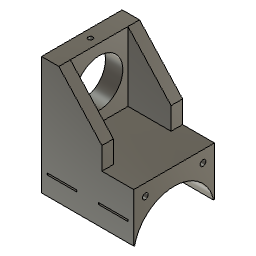
clutch holder v8 (Autodesk Fusion 360 design; units mm, degrees)
Autodesk Fusion 360 part; units mm, degrees
sketch "Sketch1" plane through (0, 0, 0) normal (0, 0, 1) x (1, 0, 0)
  line L0 (0, 0) -> (140, 0)
  line L1 (140, 0) -> (140, 140)
  line L2 (140, 140) -> (0, 140)
  line L3 (0, 140) -> (0, 0)
  line L4 (0, 140) -> (50, 140)
  line L5 (50, 140) -> (50, 0)
  line L6 (50, 0) -> (0, 0)
  line L7 (0, 0) -> (0, 140)
  dimension "d1" = 140
  dimension "d2" = 140
  constraint horizontal L0
  constraint vertical L1
  constraint horizontal L2
  constraint vertical L3
  constraint coincident L0.start L3.end
  constraint horizontal L4
  constraint vertical L5
  constraint horizontal L6
  constraint vertical L7
  constraint coincident L0 L5.end
  measures "d1" distance of L0.start L2.end
  measures "d2" distance of L0.start L0.end
extrude "Extrude1" add sketch "Sketch1" along normal blind 20 contours L0 L1 L2 L5 makes body 1
extrude "Extrude2" add sketch "Sketch1" along normal blind 140 contours L0 L2 L3 L4 L5 L6 L7 bodies 1
sketch "Sketch2" plane through (0, 0, 0) normal (-1, 0, 0) x (0, -1, 0)
  line L0 (-140, 0) -> (0, 0)
  line L1 (0, 0) -> (0, 140)
  line L2 (0, 140) -> (-140, 140)
  line L3 (-140, 140) -> (-140, 0)
  circle A0 centre (-70, 80) radius 41
  circle A1 centre (-70, 80) radius 51
  dimension "d7" = 82
  dimension "d8" = 102
  constraint concentric A0 A1
  measures "d7" diameter of A0
  measures "d8" diameter of A1
extrude "Extrude3" cut sketch "Sketch2" against normal blind 100 contours A0 bodies 1
sketch "Sketch3" plane through (0, 0, 20) normal (0, 0, 1) x (-1, 0, 0)
  line L0 (-50, -140) -> (-50, 0)
  line L1 (-50, 0) -> (-140, 0)
  line L2 (-140, 0) -> (-140, -140)
  line L3 (-140, -140) -> (-50, -140)
sketch "Sketch4" plane through (50, 0, 0) normal (1, 0, 0) x (0, 1, 0)
  circle A0 centre (70, 80) radius 41
  line L0 (0, 20) -> (140, 20)
  line L1 (140, 20) -> (140, 140)
  line L2 (140, 140) -> (0, 140)
  line L3 (0, 140) -> (0, 20)
extrude "Extrude4" cut sketch "Sketch4" against normal blind 20 bodies 1
sketch "Sketch5" plane through (0, 0, 0) normal (0, -1, 0) x (1, 0, 0)
  line L0 (30, 20) -> (30, 140)
  line L1 (30, 140) -> (0, 140)
  line L2 (0, 140) -> (0, 0)
  line L3 (0, 0) -> (140, 0)
  line L4 (140, 0) -> (140, 20)
  line L5 (140, 20) -> (30, 20)
  line L6 (30, 20) -> (30, 140)
  line L7 (140, 20) -> (30, 20)
  line L8 (30, 140) -> (140, 20)
  constraint coincident L0.end L1.start
  constraint coincident L4.end L5.start
extrude "Extrude5" add sketch "Sketch5" against normal blind 20 contours L0 L5 L6 L7 L8 bodies 1
sketch "Sketch6" plane through (0, 140, 0) normal (0, 1, 0) x (-1, 0, 0)
  line L0 (-30, 140) -> (-30, 20)
  line L1 (-30, 20) -> (-140, 20)
  line L2 (-140, 20) -> (-140, 0)
  line L3 (-140, 0) -> (0, 0)
  line L4 (0, 0) -> (0, 140)
  line L5 (0, 140) -> (-30, 140)
  line L6 (-30, 140) -> (-30, 20)
  line L7 (-140, 20) -> (-50, 20)
  line L8 (-30, 140) -> (-140, 20)
  constraint coincident L0.start L5.end
  constraint coincident L1.end L2.start
extrude "Extrude6" add sketch "Sketch6" against normal blind 20 contours L0 L1 L6 L7 L8 bodies 1
sketch "Sketch7" plane through (0, 0, 0) normal (-1, 0, 0) x (0, -1, 0)
  line L0 (-70, 80) -> (-70, 58.5)
  dimension "d17" = 21.5
  constraint vertical L0
  measures "d17" distance of L0.start L0.end
sketch "Sketch8" plane through (0, 120, 0) normal (0, -1, 0) x (1, 0, 0)
  line L0 (30, 140) -> (30, 20)
  line L1 (30, 20) -> (140, 20)
  line L2 (140, 20) -> (30, 140)
sketch "Sketch9" plane through (0, 0, 20) normal (0, 0, 1) x (-1, 0, 0)
sketch "Sketch10" plane through (0, 120, 0) normal (0, -1, 0) x (1, 0, 0)
  line L0 (104.5688, 58.4811) -> (30, 58.4811)
  line L1 (30, 58.4811) -> (30, 48.4811)
  line L2 (30, 48.4811) -> (104.5688, 48.4811)
  line L3 (104.5688, 48.4811) -> (104.5688, 58.4811)
  dimension "d18" = 10
  constraint horizontal L0
  constraint vertical L1
  constraint horizontal L2
  constraint vertical L3
  measures "d18" distance of L0.start L2.end
extrude "Extrude7" add sketch "Sketch10" along normal blind 100 bodies 1
sketch "Sketch11" plane through (104.5688, 0, 0) normal (1, 0, 0) x (0, 1, 0)
  line L0 (120, 48.4811) -> (120, 58.4811)
  line L1 (120, 58.4811) -> (20, 58.4811)
  line L2 (20, 58.4811) -> (20, 48.4811)
  line L3 (20, 48.4811) -> (120, 48.4811)
  line L4 (20, 58.4811) -> (120, 58.4811)
  line L5 (120, 58.4811) -> (120, 48.4811)
  line L6 (120, 48.4811) -> (20, 48.4811)
  line L7 (20, 48.4811) -> (20, 58.4811)
  constraint horizontal L4
  constraint vertical L5
  constraint horizontal L6
  constraint vertical L7
  constraint coincident L0.start L3.end
  constraint coincident L1.end L2.start
extrude "Extrude8" add sketch "Sketch11" along normal blind 100 bodies 1
move_face "MoveFace1" by (30, 0, 0) 1 faces at (138.0067, 86.6667, 58.4811) on bodies 1
move_face "MoveFace2" by (10, 0, 0) 1 faces at (138.0067, 86.6667, 58.4811) on bodies 1
sketch "Sketch12" plane through (0, 0, 58.4811) normal (0, 0, 1) x (-1, 0, 0)
  line L0 (-104.7257, -120) -> (-30, -120)
  line L1 (-30, -120) -> (-30, -104.8989)
  line L2 (-30, -104.8989) -> (-30, -35.1011)
  line L3 (-30, -35.1011) -> (-30, -20)
  line L4 (-30, -20) -> (-104.7257, -20)
  line L5 (-104.7257, -20) -> (-204.5688, -20)
  line L6 (-204.5688, -20) -> (-204.5688, -120)
  line L7 (-204.5688, -120) -> (-104.7257, -120)
  line L8 (-140, -20) -> (-30, -20)
  line L9 (-30, -20) -> (-30, -120)
  line L10 (-30, -120) -> (-140, -120)
  line L11 (-140, -120) -> (-140, -20)
  constraint horizontal L8
  constraint vertical L9
  constraint horizontal L10
  constraint vertical L11
  constraint coincident L0.end L1.start
  constraint coincident L5 L8.start
extrude "Extrude9" cut sketch "Sketch12" against normal blind 20 contours L0 L1 L2 L3 L4 L5 L7 L8 L9 L10 L11 bodies 1 makes body 2 at (161.5229, 86.6667, 48.4811)
sketch "Sketch13" plane through (0, 0, 20) normal (0, 0, 1) x (-1, 0, 0)
  line L0 (-140, 0) -> (-240, 0)
  line L1 (-240, 0) -> (-240, -140)
  line L2 (-240, -140) -> (-140, -140)
  line L3 (-140, -140) -> (-140, 0)
  constraint horizontal L0
  constraint vertical L1
  constraint horizontal L2
  constraint vertical L3
extrude "Extrude10" add sketch "Sketch13" along normal blind 38.5 bodies 1 2
extrude "Extrude11" add 1 faces at (206.6667, 53.3333, 20) along direction (0, 0, -1) blind 20 on bodies 1 bodies 1
sketch "Sketch14" plane through (0, 0, 0) normal (0, -1, 0) x (1, 0, 0)
  line L0 (30, 140) -> (0, 140)
  line L1 (0, 140) -> (0, 0)
  line L2 (0, 0) -> (240, 0)
  line L3 (240, 0) -> (240, 58.5)
  line L4 (240, 58.5) -> (140, 58.5)
  line L5 (140, 58.5) -> (140, 20)
  line L6 (140, 20) -> (30, 140)
  line L7 (140, 58.5) -> (104.7083, 58.5)
  constraint coincident L4.end L5.start
  constraint coincident L6 L7.end
  constraint perpendicular L5 L7
extrude "Extrude12" add sketch "Sketch14" against normal blind 20 contours L5 L6 L7 bodies 1
sketch "Sketch15" plane through (0, 140, 0) normal (0, 1, 0) x (-1, 0, 0)
  line L0 (-240, 0) -> (0, 0)
  line L1 (0, 0) -> (0, 140)
  line L2 (0, 140) -> (-30, 140)
  line L3 (-30, 140) -> (-140, 20)
  line L4 (-140, 20) -> (-140, 58.5)
  line L5 (-140, 58.5) -> (-240, 58.5)
  line L6 (-240, 58.5) -> (-240, 0)
  line L7 (-140, 58.5) -> (-104.7083, 58.5)
  constraint coincident L4.end L5.start
  constraint coincident L3 L7.end
  constraint perpendicular L4 L7
extrude "Extrude13" add sketch "Sketch15" against normal blind 20 contours L3 L4 L7 bodies 1
extrude "Extrude14" cut 1 faces at (206.6667, 86.6667, 58.5) along direction (0, 0, -1) blind 40 on bodies 1 bodies 1
extrude "Extrude15" add 1 faces at (206.6667, 86.6667, 18.5) along direction (0, 0, 1) blind 1.5 on bodies 1 bodies 1
extrude "Extrude16" cut 1 faces at (240, 46.6667, 6.6667) along direction (-1, 0, 0) blind 130 on bodies 1 bodies 1
sketch "Sketch16" plane through (0, 0, 140) normal (0, 0, 1) x (-1, 0, 0)
  line L0 (-30, 0) -> (-30, -20)
  line L1 (-30, -20) -> (-30, -120)
  line L2 (-30, -120) -> (-30, -140)
  line L3 (-30, -140) -> (0, -140)
  line L4 (0, -140) -> (0, 0)
  line L5 (0, 0) -> (-30, 0)
  circle A0 centre (-15, -70) radius 4
  dimension "d39" = 8
  measures "d39" diameter of A0
extrude "Extrude17" cut sketch "Sketch16" against normal blind 40 contours A0 bodies 1
sketch "Sketch17" plane through (0, 0, 0) normal (0, 0, -1) x (1, 0, 0)
  line L0 (110, -140) -> (110, 0)
  line L1 (110, 0) -> (0, 0)
  line L2 (0, 0) -> (0, -140)
  line L3 (0, -140) -> (110, -140)
sketch "Sketch18" plane through (0, 0, 0) normal (0, 0, 1) x (1, 0, 0)
sketch "Sketch19" plane through (0, 0, 0) normal (1, 0, 0) x (0, 1, 0)
  line L0 (0, 0) -> (140, 0)
  line L1 (140, 0) -> (140, -80)
  line L2 (0, -80) -> (0, 0)
  arc A0 (140, -80) -> (0, -80) centre (70, -80) ccw
  line L3 (138.3699, -64.9814) -> (140, -64.9814)
  line L4 (1.6301, -64.9814) -> (0, -64.9814)
  constraint horizontal L0
  constraint vertical L1
  constraint vertical L2
  constraint coincident L0.start L2.end
  constraint tangent L1 A0
  constraint coincident A0 L3.start
  constraint coincident L1 L3.end
  constraint perpendicular L1 L3
  constraint coincident A0 L4.start
  constraint coincident L2 L4.end
  constraint perpendicular L2 L4
extrude "Extrude18" add sketch "Sketch19" along normal blind 160 contours L0 L1 L2 A0 L3 L4 bodies 1
extrude "Extrude19" add 1 faces at (126.6667, 46.6667, 0) along direction (0, 0, 1) blind 20 on bodies 1 bodies 1
sketch "Sketch20" plane through (160, 0, 0) normal (1, 0, 0) x (0, 1, 0)
  line L0 (138.3699, -64.9814) -> (140, -64.9814)
  line L1 (140, -64.9814) -> (140, 20)
  line L2 (140, 20) -> (0, 20)
  line L3 (0, 20) -> (0, -64.9814)
  line L4 (0, -64.9814) -> (1.6301, -64.9814)
  arc A0 (138.3699, -64.9814) -> (1.6301, -64.9814) centre (70, -80) ccw
  circle A1 centre (20, 0) radius 5
  circle A2 centre (120, 0) radius 5
  dimension "d49" = 10
  dimension "d50" = 10
  measures "d49" diameter of A1
  measures "d50" diameter of A2
extrude "Extrude20" cut sketch "Sketch20" against normal blind 19 contours A2 bodies 1
extrude "Extrude21" cut sketch "Sketch20" against normal blind 19 contours A1 bodies 1
sketch "Sketch21" plane through (0, 0, 0) normal (0, -1, 0) x (1, 0, 0)
  line L0 (160, 20) -> (104.7083, 20)
  line L1 (104.7083, 20) -> (104.7083, 58.5)
  line L2 (104.7083, 58.5) -> (30, 140)
  line L3 (30, 140) -> (0, 140)
  line L4 (0, 140) -> (0, -64.9814)
  line L5 (0, -64.9814) -> (160, -64.9814)
  line L6 (160, -64.9814) -> (160, 20)
  line L7 (150, -30) -> (99, -30)
  line L8 (99, -30) -> (99, -33)
  line L9 (99, -33) -> (150, -33)
  line L10 (150, -33) -> (150, -30)
  line L11 (10, -30) -> (61, -30)
  line L12 (61, -30) -> (61, -33)
  line L13 (61, -33) -> (10, -33)
  line L14 (10, -33) -> (10, -30)
  dimension "d57" = 3
  dimension "d58" = 51
  constraint horizontal L7
  constraint vertical L8
  constraint horizontal L9
  constraint vertical L10
  constraint horizontal L11
  constraint vertical L12
  constraint horizontal L13
  constraint vertical L14
  measures "d57" distance of L11.start L13.end
  measures "d58" distance of L11.start L11.end
extrude "Extrude22" cut sketch "Sketch21" against normal blind 180 contours L7 L8 L9 L10 bodies 1
extrude "Extrude23" cut sketch "Sketch21" against normal blind 235 contours L11 L12 L13 L14 bodies 1
